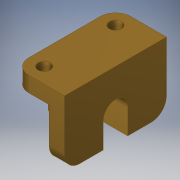
# Autodesk Inventor part: Block4
Saved by Autodesk Inventor 2019 (Build 230136000, 136)
## iProperties
Created: 2018-11-06
Part Number: Block4
Material: Brass, Soft Yellow
Document SubType Name: Modeling
Designer: 2003189
Density: 8.47 g/cm^3
Appearance: Brass - Satin
Author: 2003189
Autodesk Inventor part; units mm, degrees
ref_plane "YZ Plane" through (0, 0, 0) normal (1, 0, 0) x (0, 1, 0)
ref_plane "XZ Plane" through (0, 0, 0) normal (0, 1, 0) x (-1, 0, 0)
ref_plane "XY Plane" through (0, 0, 0) normal (0, 0, 1) x (1, 0, 0)
sketch "Sketch1" plane through (0, 0, 0) normal (0, 1, 0) x (-1, 0, 0)
  line L0 (0, 0) -> (-50, 0)
  line L1 (-50, 0) -> (-50, -100)
  line L2 (-50, -100) -> (0, -100)
  line L3 (0, -100) -> (0, 0)
  dimension "d0" = 50
  dimension "d1" = 100
  constraints: 8 end point, 2 parallel, 1 horizontal, 1 perpendicular
  measures "d0" distance of L2.end L1.end
  measures "d1" distance of L1.end L0.end
extrude "Extrusion1" add sketch "Sketch1" along normal blind 65
sketch "Sketch2" plane through (50, 0, 0) normal (1, 0, 0) x (0, 0, -1)
  line L0 (0, 0) -> (100, 0) projected
  line L1 (50, 0) -> (50, 25)
  circle A0 centre (50, 25) radius 12
  line L2 (0, 65) -> (100, 65) projected
  line L3 (50, 65) -> (50, 25)
  dimension "d5" = 24
  dimension "d15" = 40
  dimension "d16" = 40
  constraints: 4 end point, 2 midpoint, 1 centre point, 1 coincident, 1 point on line, 1 vertical
  measures "d5" diameter of A0
  measures "d15" distance of L3.start L3.end
  measures "d16" distance from line of A0.centre L2
extrude "Extrusion2" cut sketch "Sketch2" against normal blind 65
sketch "Sketch3" plane through (0, 0, -100) normal (-1, 0, 0) x (0, 0, 1)
  circle A0 centre (50, 25) radius 12 projected
  line L0 (0, 0) -> (100, 0) projected
  line L1 (62.5625, 0) -> (38, 0)
  circle A1 centre (50, 25) radius 12 projected
  line L2 (0, 0) -> (100, 0) projected
  line L3 (100, 0) -> (100, 65) projected
  line L4 (0, 65) -> (100, 65) projected
  line L5 (0, 0) -> (0, 65) projected
  line L6 (62, 25) -> (62, 0)
  line L7 (38, 25) -> (38, 0)
  line L8 (100, 0) -> (0, 0) projected
  constraints: 6 end point, 3 point on line, 2 perpendicular, 2 point on circle, 2 tangent, 1 collinear
extrude "Extrusion3" cut sketch "Sketch3" against normal blind 65 contours L6 L0 L7 A0
sketch "Sketch4" plane through (0, 0, 0) normal (0, -1, 0) x (1, 0, 0)
  line L0 (0, -100) -> (0, 0) projected
  line L1 (0, -100) -> (35, -100)
  line L2 (35, -100) -> (35, -70)
  line L3 (35, -70) -> (0, -70)
  line L4 (0, -70) -> (0, -100)
  line L5 (0, 0) -> (50, 0) projected
  line L6 (0, 0) -> (35, 0)
  line L7 (35, 0) -> (35, -30)
  line L8 (35, -30) -> (0, -30)
  line L9 (0, -30) -> (0, 0)
  dimension "d10" = 35
  dimension "d11" = 30
  dimension "d12" = 30
  constraints: 16 end point, 4 parallel, 2 horizontal, 2 perpendicular
  measures "d10" distance of L3.end L2.end
  measures "d11" distance of L2.end L1.end
  measures "d12" distance of L6.end L7.end
extrude "Extrusion4" cut sketch "Sketch4" against normal blind 50
sketch "Sketch5" plane through (0, 65, -100) normal (-1, 0, 0) x (0, 0, 1)
  line L0 (0, -15) -> (30, -15) projected
  line L1 (30, -15) -> (30, -65) projected
  line L2 (30, -65) -> (38, -65) projected
  line L3 (38, -65) -> (38, -40) projected
  arc A0 (62, -40) -> (38, -40) centre (50, -40) ccw projected
  line L4 (62, -40) -> (62, -65) projected
  line L5 (62, -65) -> (70, -65) projected
  line L6 (70, -65) -> (70, -15) projected
  line L7 (70, -15) -> (100, -15) projected
  line L8 (100, -15) -> (100, 0) projected
  line L9 (0, 0) -> (100, 0) projected
  line L10 (0, -15) -> (0, 0) projected
  line L11 (70, -15) -> (30, -15)
  point P0 (100, -65)
  constraints: 2 end point, 1 horizontal
extrude "Extrusion5" cut sketch "Sketch5" against normal blind 4 contours L11 L6 L5 L4 A0 L3 L2 L1
sketch "Sketch6" plane through (35, 0, -70) normal (0, 0, -1) x (-1, 0, 0)
  circle A0 centre (16, 15) radius 5
  line L0 (31, 0) -> (31, 50) projected
  line L1 (31, 0) -> (0, 0) projected
  point P0 (35, 0)
  dimension "d19" = 10
  dimension "d20" = 15
  dimension "d21" = 15
  constraints: 1 centre point
  measures "d19" diameter of A0
  measures "d20" distance from line of A0.centre L0
  measures "d21" distance from line of L1 A0.centre
extrude "Extrusion6" cut sketch "Sketch6" against normal through all
chamfer "Chamfer1" distance 15 angle 45 2 edges at (4, 0, -34) (4, 0, -66)
fillet "Fillet1" radius 15 4 edges at (42.5, 0, 0) (42.5, 0, -100) (0, 57.5, -100) (0, 57.5, 0)
sketch "Sketch7" plane through (0, 50, 0) normal (0, -1, 0) x (1, 0, 0)
  circle A0 centre (15, -85) radius 6
  circle A1 centre (15, -15) radius 6
  line L0 (0, -85) -> (0, -15) projected
  line L1 (15, 0) -> (35, 0) projected
  line L2 (35, -100) -> (15, -100) projected
  point P0 (0, 0)
  dimension "d28" = 12
  dimension "d29" = 12
  dimension "d30" = 15
  dimension "d31" = 15
  dimension "d32" = 15
  dimension "d33" = 15
  constraints: 2 centre point
  measures "d28" diameter of A0
  measures "d29" diameter of A1
  measures "d30" distance from line of A1.centre L0
  measures "d31" distance from line of A1.centre L1
  measures "d32" distance from line of A0.centre L2
  measures "d33" distance from line of A0.centre L0
extrude "Extrusion7" cut sketch "Sketch7" against normal through all
body "Solid1"
